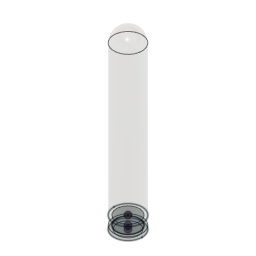
magnet-applicator-6mmx2mm (Autodesk Fusion 360 design; units mm, degrees)
Autodesk Fusion 360 part; units mm, degrees
sketch "Base - Top" plane through (0, 0, 0) normal (0, 1, 0) x (1, 0, 0)
  circle A0 centre (0, 0) radius 4
  dimension "d6" = 8
  constraint coincident A0.centre origin
  measures "d6" diameter of A0
extrude "Extrude1" add sketch "Base - Top" along normal blind 1
sketch "Cavity - Top" plane through (0, 1, 0) normal (0, 1, 0) x (-1, 0, 0)
  circle A0 centre (0, 0) radius 4
  circle A1 centre (0, 0) radius 3.25
  dimension "d9" = 6.5
  constraint coincident A0.centre A1.centre
  measures "d9" diameter of A1
extrude "Extrude2" add sketch "Cavity - Top" along normal blind 2.5
sketch "Handle - Top" plane through (0, 3.5, 0) normal (0, 1, 0) x (-1, 0, 0)
  circle A0 centre (0, 0) radius 3.25
  circle A1 centre (0, 0) radius 4
  circle A2 centre (0, 0) radius 4
  dimension "d12" = 8
  constraint coincident A0.centre A1.centre
  measures "d12" diameter of A2
extrude "Extrude3" add sketch "Handle - Top" along normal blind 46.5 contours A0 | A1 A2
fillet "Fillet1" radius 4 1 edges at (3.7293, 50, -1.4465)
fillet "Fillet2" radius 1 1 edges at (-3.7293, 0, 1.4465)
equation "full_length = 50 mm" comment "Full length of the applicator."
equation "full_width = 8 mm" comment "Full width of the applicator."
equation "cavity_depth = 1 mm" comment "Depth at which the magnet cavity begins."
equation "cavity_height = magnet_height + cavity_accuracy" comment "The height of the cavity."
equation "cavity_width = magnet_width + cavity_accuracy" comment "The width of the cavity."
equation "d6 = full_width"
equation "d7 = cavity_depth"
equation "d9 = cavity_width"
equation "d10 = cavity_height"
equation "d12 = full_width"
equation "d13 = handle_length"
equation "handle_length = full_length - cavity_height - cavity_depth" comment "Length from top of handle to top of cavity."
equation "magnet_height = 2 mm" comment "Height of the magnet."
equation "magnet_width = 6 mm" comment "Width of the magnet."
equation "cavity_accuracy = 0.5 mm" comment "How much extra space to give the magnet cavity."
equation "handle_fillet = full_width / 2" comment "Amount to fillet the top of the handle."
equation "d21 = handle_fillet"
equation "tip_fillet = 1 mm" comment "Amount to fillet the magnet-end of the applicator."
equation "d24 = tip_fillet"
